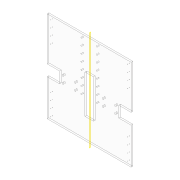
# Autodesk Inventor part: Piv Pannel 2
Saved by Autodesk Inventor 2018 (Build 220112000, 112)
## iProperties
Created: 2018-01-09
Part Number: Piv Pannel 2
Material: Polycarbonate, Clear
Document SubType Name: Modeling
Designer: dsayers
Density: 1.2 g/cm^3
Appearance: Polycarbonate - Clear
Mass: 735.163 g
Surface Area: 2051.74 cm^2
Volume: 612.636 cm^3
Author: dsayers
Autodesk Inventor part; units mm, degrees
ref_plane "YZ Plane" through (0, 0, 0) normal (1, 0, 0) x (0, 1, 0)
ref_plane "XZ Plane" through (0, 0, 0) normal (0, 1, 0) x (-1, 0, 0)
ref_plane "XY Plane" through (0, 0, 0) normal (0, 0, 1) x (1, 0, 0)
sketch "Sketch1" plane through (0, 0, 0) normal (0, 0, 1) x (1, 0, 0)
  line L0 (0, 0) -> (304.8, 0)
  line L1 (304.8, 0) -> (304.8, 330.2)
  line L2 (304.8, 330.2) -> (0, 330.2)
  line L3 (0, 330.2) -> (0, 0)
  dimension "d0" = 304.8
  dimension "d1" = 330.2
  constraints: 8 end point, 2 parallel, 1 horizontal, 1 perpendicular
  measures "d0" distance of L1.end L2.end
  measures "d1" distance of L0.end L1.end
extrude "Extrusion1" add sketch "Sketch1" along normal blind 6.35
sketch "Sketch2" plane through (0, 0, 0) normal (0, 0, -1) x (-1, 0, 0)
  line L0 (-323.0002, 172.6) -> (-260.0002, 172.6)
  line L1 (-323.0002, 132.2) -> (-260.0002, 132.2)
  line L2 (-246.7514, 152.4) -> (-364.8335, 152.4)
  line L3 (-304.8, 0) -> (-304.8, 330.2) projected
  line L4 (-304.8, 172.6) -> (-260.0002, 172.6)
  line L5 (-260.0002, 172.6) -> (-260.0002, 132.2)
  line L6 (-260.0002, 132.2) -> (-304.8, 132.2)
  line L7 (-304.8, 132.2) -> (-304.8, 172.6)
  point P0 (0, 0)
  dimension "d4" = 20.2
  dimension "d5" = 20.2
  constraints: 14 end point, 4 horizontal, 2 parallel, 2 point on line, 1 perpendicular, 4 other
  measures "d4" distance between parallel lines of L0 L2
  measures "d5" distance between parallel lines of L1 L2
extrude "Extrusion2" cut sketch "Sketch2" against normal blind 25.4
ref_plane "Work Plane1" through (152.4, 330.2, 6.35) normal (1, 0, 0) x (0, 0, -1)
mirror "Mirror1" about plane through (152.4, 330.2, 6.35) normal (1, 0, 0) of "Extrusion2"
sketch "Sketch3" plane through (0, 0, 0) normal (0, 0, -1) x (-1, 0, 0)
  circle A0 centre (-203.2502, 165.1) radius 2.0193 projected
  circle A1 centre (-247.7002, 165.1) radius 2.0193 projected
  circle A2 centre (-247.7002, 139.7) radius 2.0193 projected
  circle A3 centre (-203.2502, 139.7) radius 2.0193 projected
  circle A4 centre (-101.5498, 165.1) radius 2.0193 projected
  circle A5 centre (-101.5498, 139.7) radius 2.0193 projected
  circle A6 centre (-57.0998, 165.1) radius 2.0193 projected
  circle A7 centre (-57.0998, 139.7) radius 2.0193 projected
  point P0 (0, 0)
  constraints: 8 coincident
hole "Hole1" at (247.7002, 165.1, 0) at (203.2502, 165.1, 0) at (203.2502, 139.7, 0) at (247.7002, 139.7, 0) at (101.5498, 165.1, 0) at (101.5498, 139.7, 0) at (57.0998, 139.7, 0) at (57.0998, 165.1, 0) direction (0, 0, 1) diameter 6.35 depth 25.4 tip angle 118
sketch "Sketch4" plane through (0, 0, 0) normal (0, 0, -1) x (-1, 0, 0)
  circle A0 centre (-292.1, 317.5) radius 1.27 projected
  circle A1 centre (-292.1, 266.7) radius 1.27 projected
  circle A2 centre (-292.1, 241.3) radius 1.27 projected
  circle A3 centre (-292.1, 292.1) radius 1.27 projected
  line L0 (-302.26, 228.6) -> (-281.94, 228.6) projected
  line L1 (-281.94, 228.6) -> (-281.94, 330.2) projected
  line L2 (-302.26, 330.2) -> (-281.94, 330.2) projected
  line L3 (-302.26, 228.6) -> (-302.26, 330.2) projected
  line L4 (-281.94, 101.6) -> (-302.26, 101.6) projected
  line L5 (-302.26, 0) -> (-302.26, 101.6) projected
  line L6 (-281.94, 0) -> (-302.26, 0) projected
  line L7 (-281.94, 0) -> (-281.94, 101.6) projected
  circle A4 centre (-292.1, 63.5) radius 1.27 projected
  circle A5 centre (-292.1, 12.7) radius 1.27 projected
  circle A6 centre (-292.1, 38.1) radius 1.27 projected
  circle A7 centre (-292.1, 88.9) radius 1.27 projected
  point P0 (0, 0)
  constraints: 8 coincident
hole "Hole2" at (292.1, 317.5, 0) at (292.1, 292.1, 0) at (292.1, 266.7, 0) at (292.1, 241.3, 0) at (292.1, 88.9, 0) at (292.1, 63.5, 0) at (292.1, 38.1, 0) at (292.1, 12.7, 0) direction (0, 0, 1) diameter 1.778 depth 19.05 tip angle 118 clearance for "Flat Head Machine Screw (82)" size "#0" standard "Ansi Unified Screw Threads"
mirror "Mirror2" about plane through (152.4, 330.2, 6.35) normal (1, 0, 0) of "Hole2"
sketch "Sketch5" plane through (0, 0, 0) normal (0, 0, -1) x (-1, 0, 0)
  circle A0 centre (-124.5248, 165.1) radius 1.27 projected
  circle A1 centre (-124.5248, 215.9) radius 1.27 projected
  circle A2 centre (-124.5248, 266.7) radius 1.27 projected
  circle A3 centre (-124.5248, 317.5) radius 1.27 projected
  circle A4 centre (-124.5248, 292.1) radius 1.27 projected
  circle A5 centre (-124.5248, 241.3) radius 1.27 projected
  circle A6 centre (-124.5248, 190.5) radius 1.27 projected
  circle A7 centre (-124.5248, 139.7) radius 1.27 projected
  line L0 (-114.3648, 330.2) -> (-134.6848, 330.2) projected
  line L1 (-114.3648, 330.2) -> (-114.3648, 127) projected
  line L2 (-134.6848, 127) -> (-114.3648, 127) projected
  line L3 (-134.6848, 330.2) -> (-134.6848, 127) projected
  circle A8 centre (-180.2752, 165.1) radius 1.27 projected
  circle A9 centre (-180.2752, 215.9) radius 1.27 projected
  circle A10 centre (-180.2752, 266.7) radius 1.27 projected
  circle A11 centre (-180.2752, 317.5) radius 1.27 projected
  circle A12 centre (-180.2752, 292.1) radius 1.27 projected
  circle A13 centre (-180.2752, 241.3) radius 1.27 projected
  circle A14 centre (-180.2752, 190.5) radius 1.27 projected
  circle A15 centre (-180.2752, 139.7) radius 1.27 projected
  line L4 (-170.1152, 330.2) -> (-190.4352, 330.2) projected
  line L5 (-170.1152, 330.2) -> (-170.1152, 127) projected
  line L6 (-190.4352, 127) -> (-170.1152, 127) projected
  line L7 (-190.4352, 330.2) -> (-190.4352, 127) projected
  point P0 (0, 0)
  constraints: 16 coincident
hole "Hole3" at (180.2752, 139.7, 0) at (124.5248, 139.7, 0) at (124.5248, 165.1, 0) at (180.2752, 165.1, 0) at (180.2752, 190.5, 0) at (124.5248, 190.5, 0) at (124.5248, 215.9, 0) at (180.2752, 215.9, 0) at (124.5248, 241.3, 0) at (180.2752, 241.3, 0) at (180.2752, 266.7, 0) at (124.5248, 266.7, 0) at (124.5248, 292.1, 0) at (180.2752, 292.1, 0) at (124.5248, 317.5, 0) at (180.2752, 317.5, 0) direction (0, 0, 1) diameter 4.4958 depth 19.05 tip angle 118 clearance for "Flat Head Machine Screw (82)" size "#8" standard "Ansi Unified Screw Threads"
sketch "Sketch6" plane through (0, 0, 0) normal (0, 0, -1) x (-1, 0, 0)
  line L0 (-165.1, 175.9057) -> (-165.1, -141.7236) projected
  line L1 (-137.2248, 330.2) -> (-137.2248, 127) projected
  line L2 (-167.5752, 330.2) -> (-167.5752, 127) projected
  line L3 (-139.7, 175.9057) -> (-139.7, -141.7236) projected
  line L4 (-167.5752, 330.2) -> (-167.5752, 127) projected
  line L5 (-167.5752, 127) -> (-137.2248, 127)
  line L6 (-137.2248, 127) -> (-137.2248, 215.9)
  line L7 (-137.2248, 215.9) -> (-167.5752, 215.9)
  line L8 (-167.5752, 215.9) -> (-167.5752, 127)
  line L9 (-167.5752, 127) -> (-137.2248, 127)
  line L10 (-137.2248, 127) -> (-137.2248, 76.2)
  line L11 (-137.2248, 76.2) -> (-167.5752, 76.2)
  line L12 (-167.5752, 76.2) -> (-167.5752, 127)
  point P0 (0, 0)
  dimension "d29" = 88.9
  dimension "d31" = 50.8
  constraints: 16 end point, 4 parallel, 2 horizontal, 2 perpendicular, 1 point on line
  measures "d29" distance between parallel lines of L5 L7
  measures "d31" distance between parallel lines of L11 L5
extrude "Extrusion3" cut sketch "Sketch6" against normal blind 25.4
sketch "Sketch8" plane through (0, 0, 0) normal (0, 0, -1) x (-1, 0, 0)
  circle A0 centre (-1186.1371, 107.95) radius 1.27 projected
  circle A1 centre (-1211.5371, 107.95) radius 1.27 projected
  circle A2 centre (-1236.9371, 107.95) radius 1.27 projected
  circle A3 centre (-1262.3371, 107.95) radius 1.27 projected
  circle A4 centre (-1287.7371, 107.95) radius 1.27 projected
  circle A5 centre (-1313.1371, 107.95) radius 1.27 projected
  circle A6 centre (-1338.5371, 107.95) radius 1.27 projected
  circle A7 centre (-1363.9371, 107.95) radius 1.27 projected
  circle A8 centre (-1389.3371, 107.95) radius 1.27 projected
  circle A9 centre (-1414.7371, 107.95) radius 1.27 projected
  point P0 (0, 0)
  constraints: 10 coincident
hole "Hole4" at (1186.1371, 107.95, 0) at (1211.5371, 107.95, 0) at (1236.9371, 107.95, 0) at (1262.3371, 107.95, 0) at (1287.7371, 107.95, 0) at (1313.1371, 107.95, 0) at (1338.5371, 107.95, 0) at (1363.9371, 107.95, 0) at (1389.3371, 107.95, 0) at (1414.7371, 107.95, 0) direction (0, 0, 1) diameter 4.4958 depth 19.05 tip angle 118 clearance for "Flat Head Machine Screw (82)" size "#8" standard "Ansi Unified Screw Threads"
equation "\"d4\" = d5"
body "Solid1"
